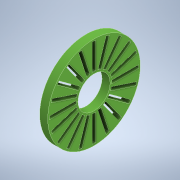
# Autodesk Inventor part: encoder
Saved by Autodesk Inventor 2021 (Build 250183000, 183)
## iProperties
Created: 2021-12-11
Part Number: encoder
Material: Generic
Document SubType Name: Modeling
Designer: Juan M. Casillas
Density: 1 g/cm^3
Appearance: Default
Author: Juan M. Casillas
Autodesk Inventor part; units mm, degrees
ref_plane "YZ Plane" through (0, 0, 0) normal (1, 0, 0) x (0, 1, 0)
ref_plane "XZ Plane" through (0, 0, 0) normal (0, 1, 0) x (-1, 0, 0)
ref_plane "XY Plane" through (0, 0, 0) normal (0, 0, 1) x (1, 0, 0)
sketch "Sketch1" plane through (0, 0, 0) normal (1, 0, 0) x (0, 1, 0)
  circle A0 centre (0, 0) radius 4
  circle A1 centre (0, 0) radius 11.5
  dimension "d0" = 8
  dimension "d1" = 23
  constraints: 2 centre point, 2 coincident
  measures "d0" diameter of A0
  measures "d1" diameter of A1
extrude "Extrusion1" add sketch "Sketch1" along normal mid plane 2
sketch "Sketch4" plane through (1, 0, 0) normal (1, 0, 0) x (0, 0, -1)
  circle A0 centre (0, 0) radius 11.5 construction
  circle A1 centre (0, 0) radius 4 construction
  line L0 (-11.5, 0) -> (-4, 0) construction
  line L1 (-11.05, -0.4) -> (-4.45, -0.4)
  line L2 (-4.45, -0.4) -> (-4.45, 0.4)
  line L3 (-4.45, 0.4) -> (-11.05, 0.4)
  line L4 (-11.05, 0.4) -> (-11.05, -0.4)
  line L5 (-11.05, -0.4) -> (-4.45, 0.4) construction
  line L6 (-4.45, -0.4) -> (-11.05, 0.4) construction
  line L7 (-4.3558, -0.9947) -> (-10.6328, -3.0342)
  line L8 (-4.1086, -1.7555) -> (-4.3558, -0.9947)
  line L9 (-10.3856, -3.7951) -> (-4.1086, -1.7555)
  line L10 (-10.6328, -3.0342) -> (-10.3856, -3.7951)
  line L11 (-3.8352, -2.292) -> (-9.1748, -6.1714)
  line L12 (-3.365, -2.9393) -> (-3.8352, -2.292)
  line L13 (-8.7045, -6.8186) -> (-3.365, -2.9393)
  line L14 (-9.1748, -6.1714) -> (-8.7045, -6.8186)
  line L15 (-2.9393, -3.365) -> (-6.8186, -8.7045)
  line L16 (-2.292, -3.8352) -> (-2.9393, -3.365)
  line L17 (-6.1714, -9.1748) -> (-2.292, -3.8352)
  line L18 (-6.8186, -8.7045) -> (-6.1714, -9.1748)
  line L19 (-1.7555, -4.1086) -> (-3.7951, -10.3856)
  line L20 (-0.9947, -4.3558) -> (-1.7555, -4.1086)
  line L21 (-3.0342, -10.6328) -> (-0.9947, -4.3558)
  line L22 (-3.7951, -10.3856) -> (-3.0342, -10.6328)
  line L23 (-0.4, -4.45) -> (-0.4, -11.05)
  line L24 (0.4, -4.45) -> (-0.4, -4.45)
  line L25 (0.4, -11.05) -> (0.4, -4.45)
  line L26 (-0.4, -11.05) -> (0.4, -11.05)
  line L27 (0.9947, -4.3558) -> (3.0342, -10.6328)
  line L28 (1.7555, -4.1086) -> (0.9947, -4.3558)
  line L29 (3.7951, -10.3856) -> (1.7555, -4.1086)
  line L30 (3.0342, -10.6328) -> (3.7951, -10.3856)
  line L31 (2.292, -3.8352) -> (6.1714, -9.1748)
  line L32 (2.9393, -3.365) -> (2.292, -3.8352)
  line L33 (6.8186, -8.7045) -> (2.9393, -3.365)
  line L34 (6.1714, -9.1748) -> (6.8186, -8.7045)
  line L35 (3.365, -2.9393) -> (8.7045, -6.8186)
  line L36 (3.8352, -2.292) -> (3.365, -2.9393)
  line L37 (9.1748, -6.1714) -> (3.8352, -2.292)
  line L38 (8.7045, -6.8186) -> (9.1748, -6.1714)
  line L39 (4.1086, -1.7555) -> (10.3856, -3.7951)
  line L40 (4.3558, -0.9947) -> (4.1086, -1.7555)
  line L41 (10.6328, -3.0342) -> (4.3558, -0.9947)
  line L42 (10.3856, -3.7951) -> (10.6328, -3.0342)
  line L43 (4.45, -0.4) -> (11.05, -0.4)
  line L44 (4.45, 0.4) -> (4.45, -0.4)
  line L45 (11.05, 0.4) -> (4.45, 0.4)
  line L46 (11.05, -0.4) -> (11.05, 0.4)
  line L47 (4.3558, 0.9947) -> (10.6328, 3.0342)
  line L48 (4.1086, 1.7555) -> (4.3558, 0.9947)
  line L49 (10.3856, 3.7951) -> (4.1086, 1.7555)
  line L50 (10.6328, 3.0342) -> (10.3856, 3.7951)
  line L51 (3.8352, 2.292) -> (9.1748, 6.1714)
  line L52 (3.365, 2.9393) -> (3.8352, 2.292)
  line L53 (8.7045, 6.8186) -> (3.365, 2.9393)
  line L54 (9.1748, 6.1714) -> (8.7045, 6.8186)
  line L55 (2.9393, 3.365) -> (6.8186, 8.7045)
  line L56 (2.292, 3.8352) -> (2.9393, 3.365)
  line L57 (6.1714, 9.1748) -> (2.292, 3.8352)
  line L58 (6.8186, 8.7045) -> (6.1714, 9.1748)
  line L59 (1.7555, 4.1086) -> (3.7951, 10.3856)
  line L60 (0.9947, 4.3558) -> (1.7555, 4.1086)
  line L61 (3.0342, 10.6328) -> (0.9947, 4.3558)
  line L62 (3.7951, 10.3856) -> (3.0342, 10.6328)
  line L63 (0.4, 4.45) -> (0.4, 11.05)
  line L64 (-0.4, 4.45) -> (0.4, 4.45)
  line L65 (-0.4, 11.05) -> (-0.4, 4.45)
  line L66 (0.4, 11.05) -> (-0.4, 11.05)
  line L67 (-0.9947, 4.3558) -> (-3.0342, 10.6328)
  line L68 (-1.7555, 4.1086) -> (-0.9947, 4.3558)
  line L69 (-3.7951, 10.3856) -> (-1.7555, 4.1086)
  line L70 (-3.0342, 10.6328) -> (-3.7951, 10.3856)
  line L71 (-2.292, 3.8352) -> (-6.1714, 9.1748)
  line L72 (-2.9393, 3.365) -> (-2.292, 3.8352)
  line L73 (-6.8186, 8.7045) -> (-2.9393, 3.365)
  line L74 (-6.1714, 9.1748) -> (-6.8186, 8.7045)
  line L75 (-3.365, 2.9393) -> (-8.7045, 6.8186)
  line L76 (-3.8352, 2.292) -> (-3.365, 2.9393)
  line L77 (-9.1748, 6.1714) -> (-3.8352, 2.292)
  line L78 (-8.7045, 6.8186) -> (-9.1748, 6.1714)
  line L79 (-4.1086, 1.7555) -> (-10.3856, 3.7951)
  line L80 (-4.3558, 0.9947) -> (-4.1086, 1.7555)
  line L81 (-10.6328, 3.0342) -> (-4.3558, 0.9947)
  line L82 (-10.3856, 3.7951) -> (-10.6328, 3.0342)
  point P0 (-7.75, 0)
  dimension "d15" = 6.6
  dimension "d16" = 0.8
  dimension "d19" = 360
  constraints: 166 end point, 3 midpoint, 2 horizontal, 2 horizontal alignment, 2 parallel, 1 coincident, 1 perpendicular, 163 other
  measures "d15" distance of L3.end L2.end
  measures "d16" distance of L2.end L1.end
extrude "Extrusion4" cut sketch "Sketch4" against normal blind 5
body "Solid1"
